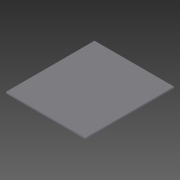
# Autodesk Inventor part: EnclosureSideLeft
Saved by Autodesk Inventor 2015 (Build 190159000, 159)
## iProperties
Created: 2014-08-22
Part Number: EnclosureSideLeft
Material: ABS Plastic
Document SubType Name: Modeling
Designer: t_clevj
Density: 1.06 g/cm^3
Appearance: Smooth - White
Author: t_clevj
Autodesk Inventor part; units mm, degrees
ref_plane "YZ Plane" through (0, 0, 0) normal (1, 0, 0) x (0, 1, 0)
ref_plane "XZ Plane" through (0, 0, 0) normal (0, 1, 0) x (-1, 0, 0)
ref_plane "XY Plane" through (0, 0, 0) normal (0, 0, 1) x (1, 0, 0)
sketch "Sketch1" plane through (0, 0, 0) normal (0, 0, 1) x (1, 0, 0)
  line L0 (-331, 20) -> (19, 20) projected
  line L1 (19, 0) -> (19, -350) projected
  line L2 (-331, -369) -> (-331, 19) projected
  line L3 (-331, -370) -> (19, -370) projected
  line L4 (19, -369) -> (19, -370) projected
  line L5 (19, -369) -> (19, -363.3) projected
  line L6 (19, -370) -> (19, 20)
  line L7 (19, 20) -> (-331, 20)
  line L8 (-331, 20) -> (-331, -370)
  line L9 (-331, -370) -> (19, -370)
  point P0 (0, 0)
  constraints: 8 end point, 2 collinear, 1 perpendicular, 1 vertical
extrude "Extrusion1" add sketch "Sketch1" along normal blind 6
body "Solid1"
